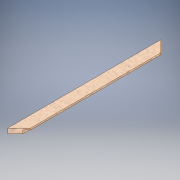
# Autodesk Inventor part: glaslat-kort
Saved by Autodesk Inventor 2019 (Build 230136000, 136)
## iProperties
Created: 2019-04-26
Part Number: glaslat-kort
Material: Generic
Document SubType Name: Modeling
Designer: Rene
Density: 1 g/cm^3
Appearance: Exterior - Beige
Author: Rene
Autodesk Inventor part; units mm, degrees
ref_plane "YZ Plane" through (0, 0, 0) normal (1, 0, 0) x (0, 1, 0)
ref_plane "XZ Plane" through (0, 0, 0) normal (0, 1, 0) x (-1, 0, 0)
ref_plane "XY Plane" through (0, 0, 0) normal (0, 0, 1) x (1, 0, 0)
sketch "Sketch1" plane through (0, 0, 0) normal (0, 0, 1) x (1, 0, 0)
  line L0 (10.5, -4.5) -> (-10.5, -4.5)
  line L1 (-10.5, -4.5) -> (-10.5, 4.5)
  line L2 (-10.5, 4.5) -> (10.5, 4.5)
  line L3 (10.5, 4.5) -> (10.5, -4.5)
  line L4 (10.5, -4.5) -> (-10.5, 4.5) construction
  line L5 (-10.5, -4.5) -> (10.5, 4.5) construction
  point P0 (0, 0)
  dimension "d0" = 21
  dimension "d1" = 9
  constraints: 12 end point, 2 midpoint, 2 parallel, 1 horizontal, 1 perpendicular
  measures "d0" distance of L0.start L0.end
  measures "d1" distance of L0.end L1.end
extrude "Extrusion1" add sketch "Sketch1" along normal mid plane 281.5
sketch "Sketch2" plane through (0, 0, 140.75) normal (0, 0, 1) x (1, 0, 0)
  line L0 (-10.5, -4.5) -> (10.5, -4.5) projected
  line L1 (10.5, -4.5) -> (3.5, -4.5)
  line L2 (3.5, -4.5) -> (3.5, 1.5)
  line L3 (3.5, 1.5) -> (10.5, 1.5)
  line L4 (10.5, 1.5) -> (10.5, -4.5)
  point P0 (0, 0)
  dimension "d4" = 6
  dimension "d5" = 7
  constraints: 8 end point, 2 parallel, 1 horizontal, 1 perpendicular
  measures "d4" distance of L1.end L2.end
  measures "d5" distance of L2.end L3.end
extrude "Extrusion2" cut sketch "Sketch2" against normal blind 282
sketch "Sketch3" plane through (-10.5, 4.5, -140.75) normal (0, 1, 0) x (1, 0, 0)
  line L0 (0, 0) -> (21, -21)
  line L1 (0, -281.5) -> (0, 0) projected
  line L2 (21, -281.5) -> (21, 0) projected
  line L3 (0, 0) -> (21, 0) projected
  point P0 (10.5, -140.75)
  dimension "d8" = 45
  constraints: 2 end point, 1 point on line, 1 other
  measures "d8" angle of L1 L0
extrude "Extrusion3" cut sketch "Sketch3" against normal blind 10
mirror "Mirror1" about plane through (0, 0, 0) normal (0, 0, 1) of "Extrusion3"
body "Solid1"
